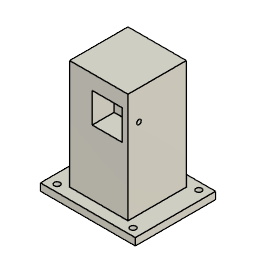
Base_Trasera (Autodesk Fusion 360 design; units mm, degrees)
Autodesk Fusion 360 part; units mm, degrees
sketch "Boceto1" plane through (0, 0, 0) normal (0, 0, 1) x (1, 0, 0)
  line L0 (0, 0) -> (40, 0)
  line L1 (40, 0) -> (40, 40)
  line L2 (40, 40) -> (0, 40)
  line L3 (0, 40) -> (0, 0)
  line L4 (52.5, -7.5) -> (-12.5, -7.5)
  line L5 (-12.5, -7.5) -> (-12.5, 47.5)
  line L6 (-12.5, 47.5) -> (52.5, 47.5)
  line L7 (52.5, 47.5) -> (52.5, -7.5)
  line L8 (52.5, -7.5) -> (-12.5, 47.5) construction
  line L9 (-12.5, -7.5) -> (52.5, 47.5) construction
  line L10 (46, -2.5) -> (-6, -2.5) construction
  line L11 (-6, -2.5) -> (-6, 42.5) construction
  line L12 (-6, 42.5) -> (46, 42.5) construction
  line L13 (46, 42.5) -> (46, -2.5) construction
  line L14 (46, -2.5) -> (-6, 42.5) construction
  line L15 (-6, -2.5) -> (46, 42.5) construction
  circle A0 centre (46, 42.5) radius 2
  circle A1 centre (-6, 42.5) radius 2
  circle A2 centre (-6, -2.5) radius 2
  circle A3 centre (46, -2.5) radius 2
  point P0 (20, 20)
  point P1 (20, 20)
  dimension "d1" = 40
  dimension "d2" = 40
  dimension "d19" = 65
  dimension "d20" = 55
  dimension "d21" = 52
  dimension "d22" = 45
  dimension "d23" = 4
  dimension "d24" = 4
  dimension "d25" = 4
  dimension "d26" = 4
  constraint horizontal L0
  constraint vertical L1
  constraint horizontal L2
  constraint vertical L3
  constraint coincident L0.start L3.end
  constraint horizontal L4
  constraint perpendicular L4 L5
  constraint parallel L4 L6
  constraint parallel L5 L7
  constraint coincident L8 P1
  constraint coincident L9 P1
  constraint horizontal L10
  constraint perpendicular L10 L11
  constraint parallel L10 L12
  constraint parallel L11 L13
  constraint coincident L14 P1
  constraint coincident L15 P1
  constraint coincident P1 P0
  constraint coincident L12.end L13.start
  constraint coincident L11.end L12.start
  constraint coincident L10.end L11.start
  constraint coincident L10.start L13.end
  measures "d1" distance of L1 L3
  measures "d2" distance of L0 L2
  measures "d19" distance of L5.end L6.end
  measures "d20" distance of L4.end L5.end
  measures "d21" distance of L11.end L12.end
  measures "d22" distance of L10.end L11.end
  measures "d23" diameter of A0
  measures "d24" diameter of A1
  measures "d25" diameter of A2
  measures "d26" diameter of A3
extrude "Extruir1" add sketch "Boceto1" along normal blind 80 contours L0 L1 L2 L3 makes body 1
sketch "Boceto2" plane through (0, 0, 0) normal (0, -1, 0) x (1, 0, 0)
  line L0 (0, 0) -> (40, 0)
  line L1 (40, 0) -> (40, 80)
  line L2 (40, 80) -> (0, 80)
  line L3 (0, 80) -> (0, 0)
  line L4 (36, 49.5) -> (15.5, 49.5)
  line L5 (15.5, 49.5) -> (15.5, 70)
  line L6 (15.5, 70) -> (36, 70)
  line L7 (36, 70) -> (36, 49.5)
  line L8 (36, 49.5) -> (15.5, 70) construction
  line L9 (15.5, 49.5) -> (36, 70) construction
  line L10 (0, 0) -> (40, 0)
  line L11 (40, 0) -> (40, 80)
  line L12 (40, 80) -> (0, 80)
  line L13 (0, 80) -> (0, 0)
  point P0 (25.75, 59.75)
  dimension "d5" = 20.5
  dimension "d6" = 20.5
  dimension "d7" = 49.5
  dimension "d8" = 4
  constraint horizontal L4
  constraint perpendicular L4 L5
  constraint parallel L4 L6
  constraint parallel L5 L7
  constraint coincident L8 P0
  constraint coincident L9 P0
  constraint horizontal L10
  constraint vertical L11
  constraint horizontal L12
  constraint vertical L13
  constraint coincident L1.end L2.start
  constraint coincident L0.start L3.end
  measures "d5" distance of L5.end L6.end
  measures "d6" distance of L4.end L5.end
  measures "d7" distance of L4 L10
  measures "d8" distance of L7 L11
extrude "Extruir2" cut sketch "Boceto2" against normal blind 15 contours L4 L5 L6 L7 bodies 1
sketch "Boceto3" plane through (0, 0, 0) normal (-1, 0, 0) x (0, -1, 0)
  line L0 (-40, 0) -> (0, 0)
  line L1 (0, 0) -> (0, 80)
  line L2 (0, 80) -> (-40, 80)
  line L3 (-40, 80) -> (-40, 0)
  line L4 (0, 0) -> (-40, 0)
  line L5 (-40, 0) -> (-40, 80)
  line L6 (-40, 80) -> (0, 80)
  line L7 (0, 80) -> (0, 0)
  line L8 (-15, 49.5) -> (-36, 49.5)
  line L9 (-36, 49.5) -> (-36, 70.5)
  line L10 (-36, 70.5) -> (-15, 70.5)
  line L11 (-15, 70.5) -> (-15, 49.5)
  line L12 (-15, 49.5) -> (-36, 70.5) construction
  line L13 (-36, 49.5) -> (-15, 70.5) construction
  point P0 (-25.5, 60)
  dimension "d11" = 21
  dimension "d12" = 21
  dimension "d13" = 49.5
  dimension "d14" = 4
  constraint horizontal L4
  constraint vertical L5
  constraint horizontal L6
  constraint vertical L7
  constraint coincident L2.end L3.start
  constraint coincident L0.end L1.start
  constraint horizontal L8
  constraint perpendicular L8 L9
  constraint parallel L8 L10
  constraint parallel L9 L11
  constraint coincident L12 P0
  constraint coincident L13 P0
  measures "d11" distance of L9.end L10.end
  measures "d12" distance of L8.end L9.end
  measures "d13" distance of L4 L8
  measures "d14" distance of L5 L9
extrude "Extruir3" cut sketch "Boceto3" against normal blind 15 contours L8 L9 L10 L11 bodies 1
sketch "Boceto4" plane through (0, 15, 0) normal (0, -1, 0) x (1, 0, 0)
  line L0 (36, 70) -> (15.5, 70)
  line L1 (15.5, 49.5) -> (36, 49.5)
  line L2 (36, 49.5) -> (36, 70)
  line L3 (15.5, 70) -> (36, 70)
  line L4 (36, 70) -> (36, 49.5)
  line L5 (36, 49.5) -> (15.5, 49.5)
  line L6 (15.5, 49.5) -> (15.5, 70)
  circle A0 centre (25.5, 60) radius 2.1
  line L7 (15.5, 70) -> (15.5, 49.5)
  dimension "d17" = 4.2
  constraint horizontal L3
  constraint vertical L4
  constraint horizontal L5
  constraint vertical L6
  constraint coincident L1.end L2.start
  constraint coincident L0.end L3.start
  measures "d17" diameter of A0
sketch "Boceto5" plane through (15, 0, 0) normal (-1, 0, 0) x (0, -1, 0)
  line L0 (-15, 70.5) -> (-36, 70.5)
  line L1 (-36, 70.5) -> (-36, 49.5)
  line L2 (-36, 49.5) -> (-15, 49.5)
  line L3 (-36, 70.5) -> (-15, 70.5)
  line L4 (-15, 70.5) -> (-15, 49.5)
  line L5 (-15, 49.5) -> (-36, 49.5)
  line L6 (-36, 49.5) -> (-36, 70.5)
  circle A0 centre (-25.5, 60) radius 2.1
  line L7 (-15, 49.5) -> (-15, 70.5)
  dimension "d18" = 4.2
  constraint horizontal L3
  constraint vertical L4
  constraint horizontal L5
  constraint vertical L6
  constraint coincident L2.end L4.end
  constraint coincident L0.end L1.start
  measures "d18" diameter of A0
extrude "Extruir4" add sketch "Boceto1" along normal blind 5 separate body makes body 2
sketch "Boceto6" plane through (40, 0, 0) normal (1, 0, 0) x (0, 1, 0)
  line L0 (0, 0) -> (40, 0)
  line L1 (40, 0) -> (40, 80)
  line L2 (40, 80) -> (0, 80)
  line L3 (0, 80) -> (0, 0)
  line L4 (0, 80) -> (0, 70)
  line L5 (0, 70) -> (15, 70)
  line L6 (15, 70) -> (15, 49.5)
  line L7 (15, 49.5) -> (0, 49.5)
  line L8 (0, 49.5) -> (0, 70)
  circle A0 centre (7.5, 59.75) radius 1.55
  dimension "d29" = 10
  dimension "d30" = 20.5
  dimension "d31" = 3.1
  constraint coincident L2.end L3.start
  constraint coincident L3 L4.end
  constraint perpendicular L2 L4
  constraint horizontal L5
  constraint vertical L6
  constraint horizontal L7
  constraint vertical L8
  measures "d29" distance of L2.end L4.end
  measures "d30" distance of L4.end L7.end
  measures "d31" diameter of A0
extrude "Extruir5" cut sketch "Boceto6" against normal blind 4 contours A0 bodies 1
sketch "Boceto7" plane through (0, 40, 0) normal (0, 1, 0) x (-1, 0, 0)
  line L0 (-40, 0) -> (0, 0)
  line L1 (0, 0) -> (0, 80)
  line L2 (0, 80) -> (-40, 80)
  line L3 (-40, 80) -> (-40, 0)
  line L4 (0, 80) -> (0, 70)
  line L5 (0, 70) -> (-15, 70)
  line L6 (-15, 70) -> (-15, 49.5)
  line L7 (-15, 49.5) -> (0, 49.5)
  line L8 (0, 49.5) -> (0, 70)
  circle A0 centre (-7.5, 59.75) radius 1.55
  dimension "d34" = 15
  dimension "d35" = 20.5
  dimension "d36" = 3.1
  constraint coincident L1.end L2.start
  constraint coincident L1 L4.end
  constraint perpendicular L2 L4
  constraint horizontal L5
  constraint vertical L6
  constraint horizontal L7
  constraint vertical L8
  measures "d34" distance of L4.end L5.end
  measures "d35" distance of L4.end L7.end
  measures "d36" diameter of A0
extrude "Extruir6" cut sketch "Boceto7" against normal blind 4 contours A0 bodies 1
